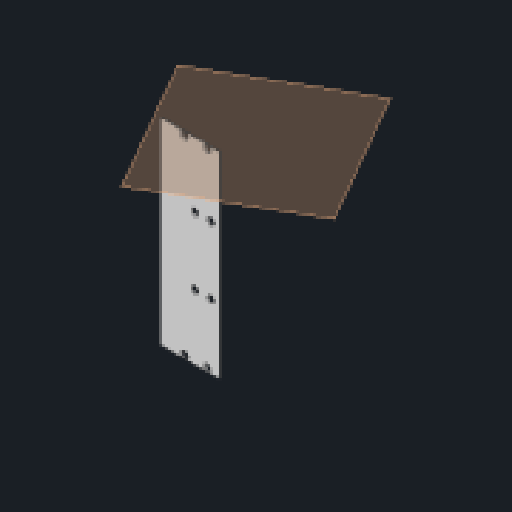
# Autodesk Inventor part: frobt
Saved by Autodesk Inventor 2023 (Build 270158000, 158)
## iProperties
Created: 2024-05-08
Part Number: frobt
Material: Generic
Document SubType Name: Modeling
Designer: szymo
Density: 1 g/cm^3
Appearance: Default
Author: szymo
Autodesk Inventor part; units mm, degrees
ref_plane "YZ Plane" through (0, 0, 0) normal (1, 0, 0) x (0, 1, 0)
ref_plane "XZ Plane" through (0, 0, 0) normal (0, 1, 0) x (-1, 0, 0)
ref_plane "XY Plane" through (0, 0, 0) normal (0, 0, 1) x (1, 0, 0)
ref_plane "Work Plane1" through (14.6553, 0, -25.7817) normal (0, 1, 0) x (-0.8660254, 0, 0.5)
sketch "Sketch1" plane through (14.6553, 0, -25.7817) normal (0, 1, 0) x (-0.8660254, 0, 0.5)
  line L0 (69.75, -10.5) -> (25.5827, 15) projected
  line L1 (69.75, -10.5) -> (69.75, -15) projected
  line L2 (69.75, -15) -> (73.75, -15) projected
  line L3 (73.75, -15) -> (73.75, -18.5) projected
  line L4 (73.75, -18.5) -> (87.75, -18.5) projected
  line L5 (87.75, -18.5) -> (73.75, -9.5) projected
  line L6 (73.75, -9.5) -> (73.75, -10.5) projected
  line L7 (73.75, -10.5) -> (69.75, -10.5) projected
  line L8 (25.5827, 15) -> (25.5827, 16)
  line L9 (25.5827, 16) -> (71.4821, -10.5)
  dimension "d0" = 1
  constraints: 4 end point, 1 parallel, 1 point on line, 1 vertical
  measures "d0" distance of L0.end L8.end
ref_plane "Work Plane2" through (-53.25, -178, -67.8971) normal (0, -1, 0) x (0.8660254, 0, -0.5)
extrude "Extrusion1" add sketch "Sketch1" against normal up to surface (178 mm away) contours L0 L8 L9 L7
sketch "Sketch2" plane through (-52.5, 0, 0.866) normal (0, 0, 1) x (1, 0, 0)
  circle A0 centre (42.0594, -3) radius 2.3 projected
  circle A1 centre (21.1782, -3) radius 2.3 projected
  circle A2 centre (30.6045, -58.5) radius 2.3 projected
  circle A3 centre (45.2015, -58.5) radius 2.3 projected
  circle A4 centre (45.2015, -119.5) radius 2.3 projected
  circle A5 centre (30.6045, -119.5) radius 2.3 projected
  circle A6 centre (21.1782, -175) radius 2.3 projected
  circle A7 centre (42.0594, -175) radius 2.3 projected
  point P0 (52.5, 0)
  constraints: 8 coincident
hole "Hole1" at (-10.4406, -3, 0.866) at (-31.3218, -3, 0.866) at (-21.8955, -58.5, 0.866) at (-7.2985, -58.5, 0.866) at (-21.8955, -119.5, 0.866) at (-7.2985, -119.5, 0.866) at (-31.3218, -175, 0.866) at (-10.4406, -175, 0.866) direction (0, 0, -1) diameter 3.6 end through all countersink diameter 6.7 countersink angle 90 clearance for "Countersunk Flat Head Screw ISO 2009/7046" size "M3" standard "ISO"
body "Solid1"
